Autodesk Fusion 360 part; units mm, degrees
note: some values were not read from the file. Set by a fixed rule: which sketch regions a step uses.
(part 2 of 2)
extrude "Extrude1''" add sketch "Sketch1 (2)" along normal blind 2 separate body contours L5 L7 L9 L11 | L7 L9 L11 A2 L12 A4 L28 L29 L30 A14 A15 | L5 L6 L7 L11 | L6 L7 L11 A2 L12 A4 L14 A5 L15 A6 L16 L17 A7 L18 A8 L19 | L8 L9 L10 A1 L13 A3 L28 L29 L30 A14 A15 | L7 L14 L16 L21 | L11 L17 L19 L20 | L14 A5 L15 A6 L16 L21 | L17 A7 L18 A8 L19 L20 | A9 | A9 L24 L25 L39 | L24 L25 L27 L39 | L24 L25 L26 L27 A12 A13 | A16 | L31 L35 L36 L38 L39 | L31 L32 L33 L34 L35 A17 A18 | L36 L37 L38 L39 A19 A20 | L39 A21 L41 L44 L46 A24 | L39 L41 L46 L47 L48 | L42 L43 A22 L45 A23 L47 L48 makes body 3 in component "versa64case_v2_bottom"
extrude "Extrude2'" add sketch "Sketch1 (2)" against normal blind 6.5 contours L5 L6 L7 L11 | L14 A5 L15 A6 L16 L21 | L17 A7 L18 A8 L19 L20 | A9 | A9 L24 L25 L39 | L24 L25 L27 L39 | L31 L35 L36 L38 L39 | L36 L37 L38 L39 A19 A20 | L39 A21 L41 L44 L46 A24 | L39 L41 L46 L47 L48 bodies 3 in component "versa64case_v2_bottom"
extrude "Extrude6''" add sketch "Sketch1 (2)" against normal blind 8.1 contours A16 bodies 3 in component "versa64case_v2_bottom"
chamfer "Chamfer2" distance 0.3 angle 45 1 edges at (31.191, 44.7498, 0) on bodies 3 in component "versa64case_v2_bottom"
extrude "Extrude7''" add sketch "Sketch1 (2)" against normal blind 6.5 contours L7 L9 L11 A2 L12 A4 L28 L29 L30 A14 A15 | L7 L14 L16 L21 | L11 L17 L19 L20 bodies 3 in component "versa64case_v2_bottom"
extrude "Extrude4''" add sketch "Sketch1 (2)" against normal blind 8.5 contours L8 L9 L10 A1 L13 A3 L28 L29 L30 A14 A15 bodies 3 in component "versa64case_v2_bottom"
extrude "Extrude5''" add sketch "Sketch1 (2)" against normal blind 8.1 contours L24 L25 L26 L27 A12 A13 | L31 L32 L33 L34 L35 A17 A18 | L42 L43 A22 L45 A23 L47 L48 bodies 3 in component "versa64case_v2_bottom"
fillet "Fillet3" radius 0.5 3 edges at (42.34, 42.75, 7.05) (31.32, 41.998, 7.05) (31.32, 45.802, 7.05) on bodies 2 in component "Versa64case_v2_top"
fillet "Fillet4" radius 0.5 8 edges at (61, 37.9, 3.6) (61, 35.9, 3.6) (61, 11.5, 3.6) (61, 9.5, 3.6) (-3, 29.3458, 3.6) (-3, 31.3458, 3.6) (-3, 11.5, 3.6) (-3, 9.5, 3.6) on bodies 2 in component "Versa64case_v2_top"
fillet "Fillet5" radius 0.5 29 edges at (-3, 4.5, 8.8) (-2.8536, 9.3536, 8.8) (29, 9.5, 8.8) (60.8536, 9.3536, 8.8) (61, 4.5, 8.8) (-2.8536, 11.6464, 8.8) (-3, 20.4229, 8.8) (-2.8536, 29.1994, 8.8) (-0.5, 29.3458, 8.8) (1.8536, 29.4922, 8.8) (2, 30.3458, 8.8) (1.8536, 31.1994, 8.8) (-0.5, 31.3458, 8.8) (-2.8536, 31.4922, 8.8) (-3, 44.6229, 8.8) (-2.8536, 57.7536, 8.8) (29, 57.9, 8.8) (60.8536, 57.7536, 8.8) (61, 47.9, 8.8) (60.8536, 38.0464, 8.8) (58.5, 37.9, 8.8) (56.1464, 37.7536, 8.8) (56, 36.9, 8.8) (56.1464, 36.0464, 8.8) (58.5, 35.9, 8.8) (60.8536, 35.7536, 8.8) (61, 23.7, 8.8) (60.8536, 11.6464, 8.8) (29, 11.5, 8.8) on bodies 2 in component "Versa64case_v2_top"
fillet "Fillet6" radius 0.5 23 edges at (0.4172, 46.9539, 8.8) (-0.0807, 40.7988, 8.8) (0.4172, 34.6437, 8.8) (8.7313, 34.1458, 8.8) (17.0454, 34.6437, 8.8) (17.5433, 40.7988, 8.8) (17.0454, 46.9539, 8.8) (8.7313, 47.4518, 8.8) (31.0649, 46.4537, 8.8) (26.0015, 43.8061, 8.8) (31.1393, 41.5114, 8.8) (32.0888, 40.4877, 8.8) (36.83, 40.21, 8.8) (41.8421, 40.7079, 8.8) (42.34, 42.08, 8.8) (42.4864, 42.6036, 8.8) (45.7882, 42.75, 8.8) (49.9384, 43.2479, 8.8) (50.4363, 45.72, 8.8) (49.9384, 48.1921, 8.8) (40.8781, 48.69, 8.8) (31.8179, 48.1921, 8.8) (31.32, 46.9398, 8.8) on bodies 2 in component "Versa64case_v2_top"
fillet "Fillet7" radius 0.5 5 edges at (-3, 0, 3.35) (-2.8536, 0, 8.6536) (29, 0, 8.8) (60.8536, 0, 8.6536) (61, 0, 3.35) on bodies 2 in component "Versa64case_v2_top"
fillet "Fillet8" radius 0.5 5 edges at (63, 0, 4.6) (62.4142, 0, 10.2142) (29, 0, 10.8) (-4.4142, 0, 10.2142) (-5, 0, 4.6) on bodies 2 in component "Versa64case_v2_top"
fillet "Fillet1'" radius 2 5 edges at (-5, 28.7, -10.1) (-4.2678, 59.1678, -10.1) (29, 59.9, -10.1) (62.2678, 59.1678, -10.1) (63, 28.7, -10.1) on bodies 3 in component "versa64case_v2_bottom"
fillet "Fillet5'" radius 0.5 8 edges at (-3, 11.5, -4.85) (-3, 29.3458, -4.85) (-3, 31.3458, -4.85) (61, 37.9, -4.85) (61, 35.9, -4.85) (61, 11.5, -4.85) (61, 9.5, -4.85) (-3, 9.5, -4.85) on bodies 3 in component "versa64case_v2_bottom"
fillet "Fillet6'" radius 0.5 29 edges at (61, 4.5, -8.1) (60.8536, 9.3536, -8.1) (29, 9.5, -8.1) (-2.8536, 9.3536, -8.1) (-3, 4.5, -8.1) (29, 11.5, -8.1) (60.8536, 11.6464, -8.1) (61, 23.7, -8.1) (60.8536, 35.7536, -8.1) (58.5, 35.9, -8.1) (56.1464, 36.0464, -8.1) (56, 36.9, -8.1) (56.1464, 37.7536, -8.1) (58.5, 37.9, -8.1) (60.8536, 38.0464, -8.1) (61, 47.9, -8.1) (60.8536, 57.7536, -8.1) (29, 57.9, -8.1) (-2.8536, 57.7536, -8.1) (-3, 44.6229, -8.1) (-2.8536, 31.4922, -8.1) (-0.5, 31.3458, -8.1) (1.8536, 31.1994, -8.1) (2, 30.3458, -8.1) (1.8536, 29.4922, -8.1) (-0.5, 29.3458, -8.1) (-2.8536, 29.1994, -8.1) (-3, 20.4229, -8.1) (-2.8536, 11.6464, -8.1) on bodies 3 in component "versa64case_v2_bottom"
fillet "Fillet7'" radius 0.5 6 edges at (25, 47.3, -8.1) (25.1464, 51.0536, -8.1) (29, 51.2, -8.1) (32.8536, 51.0536, -8.1) (33, 47.3, -8.1) (29, 39.9, -8.1) on bodies 3 in component "versa64case_v2_bottom"
chamfer "Chamfer3" distance 2 angle 45 1 edges at (30.4917, 44.4786, -10.1) on bodies 3 in component "versa64case_v2_bottom"
fillet "Fillet8'" radius 0.5 10 edges at (-5, 0, -3.85) (-4.4142, 0, -9.5142) (29, 0, -10.1) (62.4142, 0, -9.5142) (63, 0, -3.85) (61, 0, -4.6) (60.8536, 0, -7.9536) (29, 0, -8.1) (-2.8536, 0, -7.9536) (-3, 0, -4.6) on bodies 3 in component "versa64case_v2_bottom"
fillet "Fillet9" radius 0.5 16 edges at (5, 50.05, -8.1) (5.1464, 52.0536, -8.1) (9, 52.2, -8.1) (12.8536, 52.0536, -8.1) (13, 50.05, -8.1) (12.8536, 48.0464, -8.1) (9, 47.9, -8.1) (5.1464, 48.0464, -8.1) (45, 50.05, -8.1) (45.1464, 52.0536, -8.1) (49, 52.2, -8.1) (52.8536, 52.0536, -8.1) (53, 50.05, -8.1) (52.8536, 48.0464, -8.1) (49, 47.9, -8.1) (45.1464, 48.0464, -8.1) on bodies 3 in component "versa64case_v2_bottom"
sketch "Sketch1 (3)" plane through (0, 0, 10.8) normal (0, 0, 1) x (-1, 0, 0) in component "label"
  circle A0 centre (-52.9, -44.6) radius 2.75 construction
  line L0 (-1.6193, -46.7518) -> (-15.8433, -46.7518) construction
  arc A1 (-16.8433, -45.7518) -> (-15.8433, -46.7518) centre (-15.8433, -45.7518) ccw construction
  line L1 (-16.8433, -45.7518) -> (-16.8433, -35.8458) construction
  arc A2 (-15.8433, -34.8458) -> (-16.8433, -35.8458) centre (-15.8433, -35.8458) ccw construction
  line L2 (-15.8433, -34.8458) -> (-1.6193, -34.8458) construction
  arc A3 (-0.6193, -35.8458) -> (-1.6193, -34.8458) centre (-1.6193, -35.8458) ccw construction
  line L3 (-0.6193, -35.8458) -> (-0.6193, -45.7518) construction
  arc A4 (-1.6193, -46.7518) -> (-0.6193, -45.7518) centre (-1.6193, -45.7518) ccw construction
  line L4 (3, -0.5) -> (-61, -0.5) construction
  line L5 (-61, -0.5) -> (-61, -57.4) construction
  arc A5 (-61, -57.4) -> (-60.5, -57.9) centre (-60.5, -57.4) ccw construction
  line L6 (-60.5, -57.9) -> (2.5, -57.9) construction
  arc A6 (2.5, -57.9) -> (3, -57.4) centre (2.5, -57.4) ccw
  line L7 (3, -57.4) -> (3, -0.5) construction
  line L8 (-49.7363, -46.99) -> (-49.7363, -44.45) construction
  arc A7 (-48.7363, -43.45) -> (-49.7363, -44.45) centre (-48.7363, -44.45) ccw construction
  line L9 (-48.7363, -43.45) -> (-41.64, -43.45) construction
  line L10 (-41.64, -43.45) -> (-41.64, -41.91) construction
  arc A8 (-40.64, -40.91) -> (-41.64, -41.91) centre (-40.64, -41.91) ccw construction
  line L11 (-40.64, -40.91) -> (-33.02, -40.91) construction
  arc A9 (-32.02, -41.91) -> (-33.02, -40.91) centre (-33.02, -41.91) ccw construction
  line L12 (-32.02, -41.91) -> (-32.02, -46.99) construction
  arc A10 (-33.02, -47.99) -> (-32.02, -46.99) centre (-33.02, -46.99) ccw construction
  line L13 (-33.02, -47.99) -> (-48.7363, -47.99) construction
  arc A11 (-49.7363, -46.99) -> (-48.7363, -47.99) centre (-48.7363, -46.99) ccw construction
  line L14 (2.5, -56.9) -> (2.5, -1.5)
  line L15 (2, -1) -> (-60, -1)
  line L16 (-60.5, -1.5) -> (-60.5, -56.9)
  line L17 (-60, -57.4) -> (2, -57.4)
  arc A12 (-60, -1) -> (-60.5, -1.5) centre (-60, -1.5) ccw
  arc A13 (2.5, -1.5) -> (2, -1) centre (2, -1.5) ccw
  arc A14 (2, -57.4) -> (2.5, -56.9) centre (2, -56.9) ccw
  arc A15 (-60.5, -56.9) -> (-60, -57.4) centre (-60, -56.9) ccw
  arc A16 (-17.3433, -45.7518) -> (-15.8433, -47.2518) centre (-15.8433, -45.7518) ccw
  line L18 (-1.6193, -47.2518) -> (-15.8433, -47.2518)
  arc A17 (-1.6193, -47.2518) -> (-0.1193, -45.7518) centre (-1.6193, -45.7518) ccw
  line L19 (-0.1193, -35.8458) -> (-0.1193, -45.7518)
  arc A18 (-0.1193, -35.8458) -> (-1.6193, -34.3458) centre (-1.6193, -35.8458) ccw
  line L20 (-15.8433, -34.3458) -> (-1.6193, -34.3458)
  arc A19 (-15.8433, -34.3458) -> (-17.3433, -35.8458) centre (-15.8433, -35.8458) ccw
  line L21 (-17.3433, -45.7518) -> (-17.3433, -35.8458)
  line L22 (-42.64, -41.95) -> (-42.64, -41.91)
  line L23 (-2.8893, -42.7037) -> (-4.4133, -42.7037) construction
  line L24 (-5.4293, -42.7037) -> (-6.9533, -42.7037) construction
  line L25 (-7.9693, -42.7037) -> (-9.4932, -42.7037) construction
  line L26 (-10.5092, -42.7037) -> (-12.0333, -42.7037) construction
  line L27 (-13.0493, -42.7037) -> (-14.5732, -42.7037) construction
  line L28 (-34.544, -45.974) -> (-34.036, -45.974) construction
  line L29 (-37.084, -45.974) -> (-36.576, -45.974) construction
  line L30 (-39.624, -45.974) -> (-39.116, -45.974) construction
  line L31 (-42.6403, -45.974) -> (-42.1323, -45.974) construction
  line L32 (-45.1803, -45.974) -> (-44.6723, -45.974) construction
  line L33 (-47.7203, -45.974) -> (-47.2123, -45.974) construction
  circle A20 centre (-52.9, -44.6) radius 1.75 construction
  line L34 (-3.6513, -42.7037) -> (-3.6513, -47.2518) construction
  line L35 (-6.1913, -42.7037) -> (-6.1913, -47.2518) construction
  line L36 (-8.7313, -42.7037) -> (-8.7313, -47.2518) construction
  line L37 (-34.29, -45.974) -> (-34.29, -48.99) construction
  line L38 (-36.83, -45.974) -> (-36.83, -48.99) construction
  line L39 (-39.37, -45.974) -> (-39.37, -48.99) construction
  line L40 (-42.3863, -45.974) -> (-42.3863, -48.99) construction
  line L41 (-44.9263, -45.974) -> (-44.9263, -48.99) construction
  line L42 (-47.4663, -45.974) -> (-47.4663, -48.99) construction
  line L43 (-11.2713, -42.7037) -> (-11.2713, -47.2518) construction
  line L44 (-13.8113, -42.7037) -> (-13.8113, -47.2518) construction
  line L45 (-2.8893, -42.7037) -> (-3.6513, -44.0118)
  line L46 (-3.6513, -44.0118) -> (-4.4133, -42.7037)
  line L47 (-2.8893, -42.7037) -> (-4.4133, -42.7037)
  line L48 (-6.1913, -44.0118) -> (-5.4293, -42.7037)
  line L49 (-6.1913, -44.0118) -> (-6.9533, -42.7037)
  line L50 (-5.4293, -42.7037) -> (-6.9533, -42.7037)
  line L51 (-8.7313, -44.0118) -> (-7.9693, -42.7037)
  line L52 (-9.4932, -42.7037) -> (-7.9693, -42.7037)
  line L53 (-9.4932, -42.7037) -> (-8.7312, -44.0118)
  line L54 (-10.5092, -42.7037) -> (-12.0333, -42.7037)
  line L55 (-11.2713, -44.0118) -> (-10.5092, -42.7037)
  line L56 (-11.2713, -44.0118) -> (-12.0333, -42.7037)
  line L57 (-13.0493, -42.7037) -> (-13.8113, -44.0117)
  line L58 (-13.8113, -44.0117) -> (-14.5732, -42.7037)
  line L59 (-13.0493, -42.7037) -> (-14.5732, -42.7037)
  line L60 (-34.036, -45.974) -> (-34.544, -45.974)
  line L61 (-34.29, -46.4139) -> (-34.036, -45.974)
  line L62 (-34.29, -46.4139) -> (-34.544, -45.974)
  line L63 (-36.83, -46.4139) -> (-36.576, -45.974)
  line L64 (-36.576, -45.974) -> (-37.084, -45.974)
  line L65 (-37.084, -45.974) -> (-36.83, -46.4139)
  line L66 (-39.37, -46.4139) -> (-39.116, -45.974)
  line L67 (-39.116, -45.974) -> (-39.624, -45.974)
  line L68 (-39.624, -45.974) -> (-39.37, -46.4139)
  line L69 (-42.3863, -46.4139) -> (-42.1323, -45.974)
  line L70 (-42.1323, -45.974) -> (-42.6403, -45.974)
  line L71 (-42.6403, -45.974) -> (-42.3863, -46.4139)
  line L72 (-44.9263, -46.4139) -> (-44.6723, -45.974)
  line L73 (-44.6723, -45.974) -> (-45.1803, -45.974)
  line L74 (-45.1803, -45.974) -> (-44.9263, -46.4139)
  line L75 (-47.4663, -46.4139) -> (-47.2123, -45.974)
  line L76 (-47.2123, -45.974) -> (-47.7203, -45.974)
  line L77 (-47.7203, -45.974) -> (-47.4663, -46.4139)
  line L78 (-52.9, -44.6) -> (-52.9, -47.85) construction
  line L79 (-52.9, -44.6) -> (-52.2898, -43.5432)
  line L80 (-52.2898, -43.5432) -> (-53.5102, -43.5432)
  line L81 (-53.5102, -43.5432) -> (-52.9, -44.6)
  arc A21 (-33.02, -47.99) -> (-32.02, -46.99) centre (-33.02, -46.99) ccw construction
  line L82 (-48.7363, -47.99) -> (-33.02, -47.99) construction
  line L83 (-32.02, -46.99) -> (-32.02, -41.91) construction
  arc A22 (-32.02, -41.91) -> (-33.02, -40.91) centre (-33.02, -41.91) ccw construction
  line L84 (-33.02, -40.91) -> (-40.64, -40.91) construction
  arc A23 (-40.64, -40.91) -> (-41.64, -41.91) centre (-40.64, -41.91) ccw construction
  line L85 (-41.64, -41.91) -> (-41.64, -43.45) construction
  line L86 (-41.64, -43.45) -> (-48.7363, -43.45) construction
  arc A24 (-48.7363, -43.45) -> (-49.7363, -44.45) centre (-48.7363, -44.45) ccw construction
  line L87 (-49.7363, -44.45) -> (-49.7363, -46.99) construction
  arc A25 (-49.7363, -46.99) -> (-48.7363, -47.99) centre (-48.7363, -46.99) ccw construction
  circle A26 centre (-52.9, -44.6) radius 2.75 construction
  line L88 (-31.52, -41.91) -> (-31.52, -46.99)
  arc A27 (-33.02, -48.49) -> (-31.52, -46.99) centre (-33.02, -46.99) ccw
  line L89 (-33.02, -48.49) -> (-48.7363, -48.49)
  arc A28 (-50.2363, -46.99) -> (-48.7363, -48.49) centre (-48.7363, -46.99) ccw
  arc A29 (-48.7363, -42.95) -> (-49.4411, -43.1259) centre (-48.7363, -44.45) ccw
  line L90 (-48.7363, -42.95) -> (-42.64, -42.95)
  line L91 (-42.14, -42.45) -> (-42.14, -41.91)
  arc A30 (-40.64, -40.41) -> (-42.14, -41.91) centre (-40.64, -41.91) ccw
  line L92 (-40.64, -40.41) -> (-33.02, -40.41)
  arc A31 (-31.52, -41.91) -> (-33.02, -40.41) centre (-33.02, -41.91) ccw
  arc A32 (-50.1059, -42.9399) -> (-50.5791, -46.8751) centre (-52.9, -44.6) ccw
  line L93 (-50.2363, -46.99) -> (-50.2363, -47.0151)
  arc A33 (-50.2363, -47.0151) -> (-50.5791, -46.8751) centre (-50.4363, -47.0151) ccw
  arc A34 (-50.1059, -42.9399) -> (-49.4411, -43.1259) centre (-49.6761, -42.6846) ccw
  arc A35 (-42.64, -42.95) -> (-42.14, -42.45) centre (-42.64, -42.45) ccw
  dimension "d220" = 0.5
  dimension "d221" = -0.5
  dimension "d228" = 120
  dimension "d229" = 60
  dimension "d232" = 0.2
  dimension "d233" = 0.5
  dimension "d234" = 0.5
  constraint tangent L15 A12
  constraint tangent L16 A12
  constraint tangent L14 A13
  constraint tangent L15 A13
  constraint equal A12 A13
  constraint tangent L14 A14
  constraint tangent L17 A14
  constraint equal A12 A14
  constraint tangent L16 A15
  constraint tangent L17 A15
  constraint equal A12 A15
  constraint midpoint L23 L34.start
  constraint coincident L18 L34.end
  constraint perpendicular L18 L34
  constraint midpoint L24 L35.start
  constraint coincident L18 L35.end
  constraint perpendicular L18 L35
  constraint midpoint L25 L36.start
  constraint midpoint L18 L36.end
  constraint midpoint L28 L37.start
  constraint midpoint L29 L38.start
  constraint perpendicular L13 L38
  constraint midpoint L30 L39.start
  constraint midpoint L31 L40.start
  constraint midpoint L32 L41.start
  constraint midpoint L33 L42.start
  constraint midpoint L26 L43.start
  constraint coincident L18 L43.end
  constraint perpendicular L18 L43
  constraint midpoint L27 L44.start
  constraint coincident L18 L44.end
  constraint perpendicular L18 L44
  constraint coincident L23.start L45.start
  constraint coincident L34 L45.end
  constraint coincident L23.end L46.end
  constraint coincident L35 L48.start
  constraint coincident L24.start L48.end
  constraint parallel L45 L48
  constraint coincident L24.end L49.end
  constraint perpendicular L35 L50
  constraint coincident L25.start L51.end
  constraint coincident L25.end L52.start
  constraint coincident L26.start L54.start
  constraint coincident L26.end L54.end
  constraint coincident L43 L55.start
  constraint coincident L27.start L57.start
  constraint coincident L44 L57.end
  constraint parallel L55 L57
  constraint coincident L27.end L58.end
  constraint coincident L28.end L60.start
  constraint coincident L28.start L60.end
  constraint coincident L37 L61.start
  constraint coincident L38 L63.start
  constraint coincident L29.end L63.end
  constraint coincident L29.start L64.end
  constraint parallel L62 L65
  constraint coincident L39 L66.start
  constraint coincident L30.end L66.end
  constraint coincident L30.start L67.end
  constraint coincident L40 L69.start
  constraint coincident L31.end L69.end
  constraint parallel L66 L69
  constraint coincident L31.start L70.end
  constraint coincident L41 L72.start
  constraint coincident L32.end L72.end
  constraint parallel L69 L72
  constraint coincident L32.start L73.end
  constraint coincident L42 L75.start
  constraint coincident L33.end L75.end
  constraint parallel L72 L75
  constraint coincident L33.start L76.end
  constraint coincident A0.centre A20.centre
  constraint parallel L42 L78
  constraint horizontal L80
  constraint symmetric L78 L79 L81
  constraint concentric A0 A32
  constraint concentric A10 A27
  constraint concentric A11 A28
  constraint concentric A7 A29
  constraint concentric A8 A30
  constraint concentric A9 A31
  constraint tangent L88 A27
  constraint tangent L88 A31
  constraint tangent A28 L93
  constraint tangent A27 L89
  constraint tangent L89 A28
  constraint tangent A29 L90
  constraint tangent A29 L93
  constraint tangent L91 A30
  constraint tangent A30 L92
  constraint tangent L92 A31
  constraint tangent L93 A33
  constraint tangent A32 A33
  constraint tangent A29 A34
  constraint tangent A32 A34
  constraint tangent L90 A35
  constraint tangent L91 A35
  measures "d220" radius of A12
  measures "d228" angle of L60 L61
  measures "d229" angle of L79 L81
  measures "d232" radius of A33
  measures "d233" radius of A34
  measures "d234" radius of A35
extrude "Extrude1'''" add sketch "Sketch1 (3)" along normal blind 0.1 separate body makes body 4 at (44.9263, 46.1206, 10.8) makes body 5 at (34.29, 46.1206, 10.8) makes body 6 at (6.1913, 43.1397, 10.8) makes body 7 at (3.6513, 43.1397, 10.8) makes body 8 at (13.8113, 43.1397, 10.8) makes body 9 at (42.3863, 46.1206, 10.8) makes body 10 at (47.4663, 46.1206, 10.8) makes body 11 at (36.83, 46.1206, 10.8) makes body 12 at (8.7313, 43.1397, 10.8) makes body 13 at (24.8221, 12.1605, 10.8) makes body 14 at (11.2713, 43.1397, 10.8) makes body 15 at (39.37, 46.1206, 10.8) makes body 16 at (52.9, 43.8954, 10.8) in component "label"
component "Versa64cart_v1.6" placed x (1, 0, 0) y (0, 1, 0) z (0, 0, 1) at (0, 0, 0)
component "Versa64case_v2_top" placed x (1, 0, 0) y (0, 1, 0) z (0, 0, 1) at (0, 0, 0)
component "versa64case_v2_bottom" placed x (1, 0, 0) y (0, 1, 0) z (0, 0, 1) at (0, 0, 0)
component "label" placed x (1, 0, 0) y (0, 1, 0) z (0, 0, 1) at (0, 0, 0)
equation "pcb = 1.6 mm"
equation "d2 = -pcb"
equation "d4 = dipsw"
equation "d8 = dipsw + 1.7 mm"
equation "d10 = dipsw - 0.8 mm"
equation "d16 = switch_body"
equation "d18 = switch_body + 0.2 mm"
equation "stem = 12.5 mm"
equation "switch_body = 4.5 mm"
equation "d22 = stem"
equation "dipsw = 5.3 mm"
equation "socket = 4.3 mm"
equation "EPROM = 9.0 mm"
equation "d35 = socket"
equation "d37 = socket"
equation "d38 = EPROM - socket"
equation "above = 8.8 mm"
equation "d42 = above"
equation "below = 6.5 mm"
equation "dside = 3.0 mm"
equation "d45 = dside"
equation "d46 = dside"
equation "dback = 9 mm"
equation "d48 = dback"
equation "ttol = 0.5 mm"
equation "d50 = ttol"
equation "d51 = ttol"
equation "d53 = ttol"
equation "d54 = ttol"
equation "d55 = ttol"
equation "d56 = ttol"
equation "d57 = ttol"
equation "d58 = ttol"
equation "wall = 2 mm"
equation "d60 = ttol"
equation "d61 = ttol"
equation "d62 = ttol"
equation "d63 = ttol"
equation "d64 = ttol"
equation "d65 = ttol"
equation "d66 = ttol"
equation "d67 = ttol"
equation "d68 = ttol"
equation "d71 = ttol"
equation "standoff_top_dia = 6 mm"
equation "d75 = standoff_top_dia"
equation "d76 = ttol"
equation "d77 = ttol"
equation "d78 = ttol"
equation "d79 = ttol"
equation "d80 = ttol"
equation "d81 = ttol"
equation "d82 = ttol"
equation "d83 = ttol"
equation "iwall = 1.2 mm"
equation "portlen = 9.5 mm"
equation "d87 = portlen"
equation "d88 = -iwall"
equation "d89 = -iwall"
equation "d90 = icorner"
equation "d91 = icorner"
equation "icorner = 0.5 mm"
equation "d93 = swall"
equation "d94 = swall"
equation "d95 = swall"
equation "d96 = icorner + swall"
equation "d97 = icorner + swall"
equation "d98 = wall"
equation "d99 = wall"
equation "d104 = wall"
equation "d105 = wall"
equation "d110 = below"
equation "btol = 0.3 mm"
equation "d114 = btol"
equation "d115 = btol"
equation "standoff_bot_dia = 8 mm"
equation "d117 = standoff_bot_dia"
equation "d119 = btol"
equation "d120 = wall"
equation "d123 = wall"
equation "d125 = btol"
equation "d128 = -above"
equation "d130 = -above"
equation "d132 = -above + dipsw"
equation "d134 = -above - pcb"
equation "offset = 2 mm"
equation "d137 = -above - pcb + offset"
equation "d139 = wall / 2"
equation "d141 = btol"
equation "d142 = btol"
equation "d148 = wall"
equation "d150 = -below"
equation "d154 = -below - offset"
equation "d156 = -below - pcb"
equation "d158 = btol"
equation "d159 = btol"
equation "swall = 2.0 mm"
equation "d183 = swall * ofac"
equation "d184 = swall * ofac"
equation "d185 = wall"
equation "d187 = swall * ofac"
equation "d188 = swall * ofac"
equation "d189 = swall * ofac"
equation "d190 = icorner + swall * 0.6"
equation "d191 = icorner + swall * 0.6"
equation "d193 = -below - pcb"
equation "d196 = -below"
equation "d210 = btol"
equation "ofac = 0.43"
named bodies: "versa64cart"
